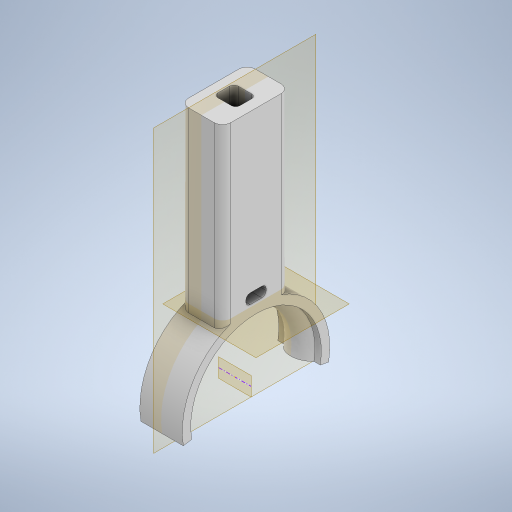
# Autodesk Inventor part: 막대4
Saved by Autodesk Inventor 2023 (Build 270158000, 158)
## iProperties
Created: 2023-04-26
Part Number: 막대4
Material: 일반
Document SubType Name: Modeling
Designer: rlatk
Density: 1 g/cm^3
Appearance: 기본값
Author: rlatk
Autodesk Inventor part; units mm, degrees
ref_plane "XZ Plane" through (0, 0, 0) normal (0, 1, 0) x (-1, 0, 0)
ref_plane "작업 평면1" through (0, 0, 11.4) normal (0, 0, 1) x (1, 0, 0)
sketch "스케치2" plane through (0, 0, 11.4) normal (0, 0, 1) x (1, 0, 0)
  line L0 (-3.8254, 0) -> (3.8254, 0)
  point P0 (0, 0)
  constraints: 2 end point, 1 horizontal
sketch "스케치1" plane through (0, 0, 0) normal (0, 1, 0) x (-1, 0, 0)
  line L0 (0, -4) -> (3.5, -4)
  line L1 (3.5, -4) -> (-3.5, -4)
  arc A0 (3.5, -4) -> (-3.5, -4) centre (0, -5.9365) ccw
  line L2 (0, -9.48) -> (0, 14.88) projected
  line L3 (0, -4) -> (0, -6)
  line L4 (0, -6) -> (5, -6)
  line L5 (5, -6) -> (5, -4)
  line L6 (5, -4) -> (3.5, -4)
  line L7 (0, -4) -> (-5, -4)
  line L8 (-5, -4) -> (-5, -6)
  line L9 (-5, -6) -> (0, -6)
  point P0 (0, -1.9365)
  point P1 (-3.5, -4)
  dimension "d0" = 3.5
  dimension "d1" = 3.5
  dimension "d2" = 4
  dimension "d60" = 2
  dimension "d61" = 5
  dimension "d62" = 2
  dimension "d63" = 5
  dimension "d64" = 2
  constraints: 18 end point, 3 perpendicular, 3 point on circle, 2 point on line, 1 centre point, 1 collinear, 1 midpoint, 1 parallel
  measures "d0" distance of L0.start L0.end
  measures "d1" distance of L0.start L1.end
  measures "d2" radius of A0
  measures "d60" distance of L3.start L3.end
  measures "d61" distance of L3.end L4.end
  measures "d62" distance of L4.end L5.end
  measures "d63" distance of L3.start L7.end
  measures "d64" distance of L7.end L8.end
revolve "회전1" add sketch "스케치1" angle 190 about axis through (-3.8254, 0, 11.4) along (1, 0, 0) and the other way 10
ref_plane "작업 평면4" through (5, 17.4, 11.4) normal (0, 1, 0) x (-1, 0, 0)
sketch "스케치16" plane through (5, 17.4, 11.4) normal (0, 1, 0) x (-1, 0, 0)
  line L0 (10, 17.4) -> (10, -17.4) projected
  line L1 (0, 17.4) -> (0, -17.4) projected
  line L2 (0, 15.4) -> (0, -15.4) projected
  line L3 (10, -7.9) -> (0, -7.9)
  line L4 (0, -7.9) -> (0, 7.9)
  line L5 (0, 7.9) -> (10, 7.9)
  line L6 (10, 7.9) -> (10, -7.9)
  line L7 (-2, 0) -> (12, 0) projected
  point P0 (5, -11.4)
  point P1 (10, -17.1357)
  point P2 (10, 17.1357)
  point P3 (0, -17.1357)
  point P4 (0, 17.1357)
  point P5 (0, -15.166)
  point P6 (0, 15.166)
  point P7 (5, 7.9)
  point P8 (0, -7.9)
  point P9 (10, 7.9)
  point P10 (0, 7.9)
  dimension "d90" = 7.9
  dimension "d91" = 7.9
  constraints: 8 end point, 2 parallel, 2 point on line, 1 horizontal, 1 midpoint, 1 perpendicular
  measures "d90" distance from line of L7 point (5, 7.9)
  measures "d91" distance between parallel lines of L7 L3
extrude "돌출16" add sketch "스케치16" along normal blind 40
sketch "스케치17" plane through (0, 0, 0) normal (1, 0, 0) x (0, 1, 0)
  arc A0 (17.4, 11.4) -> (-3.0215, 28.5357) centre (0, 11.4) ccw projected
  arc A1 (-3.0215, -5.7357) -> (17.4, 11.4) centre (0, 11.4) ccw projected
  line L0 (17.4, 42.0558) -> (17.4, -19.2558) projected
  line L1 (17.4, 11.4) -> (17.4, 19.3) projected
  line L2 (17.4, 19.3) -> (17.4, 11.4)
  line L3 (17.4, 3.5) -> (17.4, 11.4) projected
  line L4 (17.4, 11.4) -> (17.4, 3.5)
  line L5 (17.4, 3.5) -> (15.5032, 3.5)
  line L6 (17.4, 19.3) -> (15.5032, 19.3)
  arc A2 (17.4, 11.4) -> (15.5032, 19.3) centre (0, 11.4) ccw
  arc A3 (15.5032, 3.5) -> (17.4, 11.4) centre (0, 11.4) ccw
  point P0 (0, 0)
  constraints: 8 end point, 6 point on circle, 2 centre point, 2 collinear, 2 concentric, 1 parallel, 1 perpendicular, 1 tangent
extrude "돌출17" add sketch "스케치17" along normal blind 5 and the other way blind 5
sketch "스케치18" plane through (5, 57.4, 11.4) normal (0, 1, 0) x (1, 0, 0)
  line L0 (-10, -7.9) -> (0, -7.9) projected
  line L1 (0, -7.9) -> (0, 7.9) projected
  line L2 (-10, 7.9) -> (-10, -7.9) projected
  line L3 (0, 7.9) -> (-10, 7.9) projected
  line L4 (0, -7.9) -> (-10, -7.9) projected
  line L5 (-10, 7.9) -> (0, 7.9) projected
  line L6 (-2, -7.9) -> (-8, -7.9)
  line L7 (-10, -5.9) -> (-10, 5.9)
  line L8 (-8, 7.9) -> (-2, 7.9)
  line L9 (0, 5.9) -> (0, -5.9)
  line L10 (-2.4, -1.4) -> (-2.4, 1.4)
  line L11 (-7.6, 1.4) -> (-7.6, -1.4)
  line L12 (-6.6, -2.4) -> (-3.4, -2.4)
  line L13 (-3.4, 2.4) -> (-6.6, 2.4)
  arc A0 (-2, -7.9) -> (0, -5.9) centre (-2, -5.9) ccw
  arc A1 (0, 5.9) -> (-2, 7.9) centre (-2, 5.9) ccw
  arc A2 (-8, 7.9) -> (-10, 5.9) centre (-8, 5.9) ccw
  arc A3 (-10, -5.9) -> (-8, -7.9) centre (-8, -5.9) ccw
  arc A4 (-3.4, -2.4) -> (-2.4, -1.4) centre (-3.4, -1.4) ccw
  arc A5 (-2.4, 1.4) -> (-3.4, 2.4) centre (-3.4, 1.4) ccw
  arc A6 (-6.6, 2.4) -> (-7.6, 1.4) centre (-6.6, 1.4) ccw
  arc A7 (-7.6, -1.4) -> (-6.6, -2.4) centre (-6.6, -1.4) ccw
  point P0 (-5, 11.4)
  dimension "d98" = 2.4
  dimension "d99" = 2.4
  dimension "d100" = 5.5
  dimension "d101" = 5.5
  dimension "d102" = 2
  dimension "d103" = 1
  constraints: 16 end point, 16 point on circle, 16 tangent, 8 centre point, 6 equal radius, 6 parallel, 4 point on line, 1 horizontal, 1 perpendicular
  measures "d98" distance between parallel lines of L1 L10
  measures "d99" distance between parallel lines of L2 L11
  measures "d100" distance between parallel lines of L0 L12
  measures "d101" distance between parallel lines of L3 L13
  measures "d102" radius of A0
  measures "d103" radius of A4
extrude "돌출18" cut sketch "스케치18" against normal blind 50 contours A4 L12 A7 L11 A6 L13 A5 L10
fillet "모깎기4" radius 2 4 edges at (5, 36.4516, 19.3) (5, 36.4516, 3.5) (-5, 36.4516, 3.5) (-5, 36.4516, 19.3)
sketch "스케치19" plane through (5, 0, 11.4) normal (1, 0, 0) x (0, 0, -1)
  line L0 (2.4, 57.4) -> (2.4, 13.4581) projected
  line L1 (-2.4, 57.4) -> (-2.4, 13.4581) projected
  line L2 (1.4, 17.948) -> (-1.4, 17.948)
  line L3 (-2.4, 18.948) -> (-2.4, 19.348)
  line L4 (-1.4, 20.348) -> (1.4, 20.348)
  line L5 (2.4, 19.348) -> (2.4, 18.948)
  arc A0 (1.4, 17.948) -> (2.4, 18.948) centre (1.4, 18.948) ccw
  arc A1 (2.4, 19.348) -> (1.4, 20.348) centre (1.4, 19.348) ccw
  arc A2 (-2.4, 18.948) -> (-1.4, 17.948) centre (-1.4, 18.948) ccw
  arc A3 (-1.4, 20.348) -> (-2.4, 19.348) centre (-1.4, 19.348) ccw
  point P0 (11.4, 0)
  point P1 (2.4, 17.948)
  point P2 (-2.4, 20.348)
  point P3 (0, 20.348)
  point P4 (0, 17.948)
  point P5 (2.4, 18.948)
  point P6 (2.4, 19.348)
  point P7 (-2.4, 19.348)
  point P8 (-2.4, 18.948)
  dimension "d107" = 2.4
  dimension "d108" = 1
  dimension "d109" = 1
  constraints: 8 end point, 8 point on circle, 8 tangent, 6 point on line, 4 centre point, 2 equal radius, 2 midpoint, 2 parallel, 1 horizontal, 1 perpendicular
  measures "d107" distance of point (0, 20.348) point (0, 17.948)
  measures "d108" radius of A0
  measures "d109" radius of A2
extrude "돌출19" cut sketch "스케치19" against normal blind 6
